Autodesk Inventor part; units mm, degrees
(part 4 of 4)
sketch "Sketch22" plane through (0, 0, 1.6) normal (0, 0, 1) x (1, 0, 0)
  line L0 (-10.5, 33.5) -> (-70.5, 33.5) projected
  line L1 (-70.5, 33.5) -> (-70.5, 17.8589) projected
  arc A0 (-71.1087, 16.5323) -> (-70.5, 17.8589) centre (-72.25, 17.8589) ccw projected
  arc A1 (-71.1087, 16.5323) -> (-71.1087, 10.4677) centre (-68.5, 13.5) ccw projected
  arc A2 (-70.5, 9.1411) -> (-71.1087, 10.4677) centre (-72.25, 9.1411) ccw projected
  line L2 (-70.5, 9.1411) -> (-70.5, 3) projected
  line L3 (-70.5, 3) -> (-53.1906, 3) projected
  line L4 (-53.1906, 3) -> (-51.7472, 0.5) projected
  arc A3 (-51.7472, -2.5) -> (-51.7472, 0.5) centre (-54.3453, -1) ccw projected
  line L5 (-51.7472, -2.5) -> (-53.1906, -5) projected
  line L6 (-53.1906, -5) -> (-70.5, -5) projected
  line L7 (-70.5, -5) -> (-70.5, -10.5) projected
  arc A4 (-71.3276, -12.569) -> (-70.5, -10.5) centre (-73.5, -10.5) ccw projected
  arc A5 (-71.3276, -12.569) -> (-71.3276, -28.431) centre (-63, -20.5) ccw projected
  arc A6 (-70.5, -30.5) -> (-71.3276, -28.431) centre (-73.5, -30.5) ccw projected
  line L8 (-70.5, -30.5) -> (-70.5, -37.5) projected
  line L9 (-70.5, -37.5) -> (-56.7679, -37.5) projected
  line L10 (-56.7679, -37.5) -> (-55.6132, -39.5) projected
  arc A7 (-55.6132, -41.5) -> (-55.6132, -39.5) centre (-57.3453, -40.5) ccw projected
  line L11 (-55.6132, -41.5) -> (-56.7679, -43.5) projected
  line L12 (-56.7679, -43.5) -> (-70.5, -43.5) projected
  line L13 (-70.5, -43.5) -> (-70.5, -47.4689) projected
  arc A8 (-70.5, -47.4689) -> (-69.0556, -48.3647) centre (-69.5, -47.4689) ccw projected
  arc A9 (-64.3647, -53.0556) -> (-69.0556, -48.3647) centre (-67.5, -51.5) ccw projected
  arc A10 (-64.3647, -53.0556) -> (-63.4689, -54.5) centre (-63.4689, -53.5) ccw projected
  line L14 (-63.4689, -54.5) -> (-47, -54.5) projected
  line L15 (-47, -54.5) -> (-47, -50) projected
  arc A11 (-45, -48) -> (-47, -50) centre (-45, -50) ccw projected
  line L16 (-45, -48) -> (24, -48) projected
  arc A12 (26, -50) -> (24, -48) centre (24, -50) ccw projected
  line L17 (26, -50) -> (26, -54.5) projected
  line L18 (26, -54.5) -> (63.4689, -54.5) projected
  arc A13 (63.4689, -54.5) -> (64.3647, -53.0556) centre (63.4689, -53.5) ccw projected
  arc A14 (69.0556, -48.3647) -> (64.3647, -53.0556) centre (67.5, -51.5) ccw projected
  arc A15 (69.0556, -48.3647) -> (70.5, -47.4689) centre (69.5, -47.4689) ccw projected
  line L19 (70.5, -47.4689) -> (70.5, -43.5) projected
  line L20 (70.5, -43.5) -> (57.2321, -43.5) projected
  line L21 (57.2321, -43.5) -> (58.5311, -41.25) projected
  arc A16 (58.5311, -41.25) -> (58.5311, -39.75) centre (57.2321, -40.5) ccw projected
  line L22 (58.5311, -39.75) -> (57.2321, -37.5) projected
  line L23 (57.2321, -37.5) -> (70.5, -37.5) projected
  line L24 (70.5, -37.5) -> (70.5, -30.5) projected
  arc A17 (71.3276, -28.431) -> (70.5, -30.5) centre (73.5, -30.5) ccw projected
  arc A18 (71.3276, -28.431) -> (71.3276, -12.569) centre (63, -20.5) ccw projected
  arc A19 (70.5, -10.5) -> (71.3276, -12.569) centre (73.5, -10.5) ccw projected
  line L25 (70.5, -10.5) -> (70.5, 9.6199) projected
  arc A20 (71, 10.9428) -> (70.5, 9.6199) centre (72.5, 9.6199) ccw projected
  arc A21 (71, 10.9428) -> (72.25, 14.25) centre (67.25, 14.25) ccw projected
  line L26 (72.25, 14.25) -> (72.25, 43.95) projected
  arc A22 (72.25, 43.95) -> (71, 47.2572) centre (67.25, 43.95) ccw projected
  arc A23 (70.6186, 47.9015) -> (71, 47.2572) centre (72.5, 48.5801) ccw projected
  arc A24 (70.6186, 47.9015) -> (69.194, 48.4372) centre (69.678, 47.5622) ccw projected
  arc A25 (64.3647, 53.0556) -> (69.194, 48.4372) centre (67.5, 51.5) ccw projected
  arc A26 (64.3647, 53.0556) -> (63.4689, 54.5) centre (63.4689, 53.5) ccw projected
  line L27 (63.4689, 54.5) -> (-63.4689, 54.5) projected
  arc A27 (-63.4689, 54.5) -> (-64.3647, 53.0556) centre (-63.4689, 53.5) ccw projected
  arc A28 (-69.0556, 48.3647) -> (-64.3647, 53.0556) centre (-67.5, 51.5) ccw projected
  arc A29 (-69.0556, 48.3647) -> (-70.5, 47.4689) centre (-69.5, 47.4689) ccw projected
  line L28 (-70.5, 47.4689) -> (-70.5, 39.5) projected
  line L29 (-70.5, 39.5) -> (-10.5, 39.5) projected
  arc A30 (-10.5, 33.5) -> (-10.5, 39.5) centre (-10.5, 36.5) ccw projected
  line L30 (33.5, 22.1) -> (33.5, 39.1) projected
  arc A31 (33.9581, 40.3738) -> (33.5, 39.1) centre (35.5, 39.1) ccw projected
  arc A32 (33.9581, 40.3738) -> (34.4469, 40.1682) centre (35.75, 43.95) ccw projected
  arc A33 (34.4469, 40.1682) -> (34, 39.1) centre (35.5, 39.1) ccw projected
  line L31 (34, 39.1) -> (34, 22.1) projected
  arc A34 (34, 22.1) -> (35.5, 20.6) centre (35.5, 22.1) ccw projected
  line L32 (35.5, 20.6) -> (67.5, 20.6) projected
  arc A35 (67.5, 20.6) -> (69, 22.1) centre (67.5, 22.1) ccw projected
  line L33 (69, 22.1) -> (69, 39.1) projected
  arc A36 (69, 39.1) -> (68.5531, 40.1682) centre (67.5, 39.1) ccw projected
  arc A37 (68.5531, 40.1682) -> (69.0419, 40.3738) centre (67.25, 43.95) ccw projected
  arc A38 (69.5, 39.1) -> (69.0419, 40.3738) centre (67.5, 39.1) ccw projected
  line L34 (69.5, 39.1) -> (69.5, 22.1) projected
  arc A39 (67.5, 20.1) -> (69.5, 22.1) centre (67.5, 22.1) ccw projected
  line L35 (67.5, 20.1) -> (35.5, 20.1) projected
  arc A40 (33.5, 22.1) -> (35.5, 20.1) centre (35.5, 22.1) ccw projected
  arc A41 (70.5, 39.1) -> (69.8755, 40.9322) centre (67.5, 39.1) ccw projected
  line L36 (70.5, 39.1) -> (70.5, 22.1) projected
  arc A42 (67.5, 19.1) -> (70.5, 22.1) centre (67.5, 22.1) ccw projected
  line L37 (67.5, 19.1) -> (35.5, 19.1) projected
  arc A43 (32.5, 22.1) -> (35.5, 19.1) centre (35.5, 22.1) ccw projected
  line L38 (32.5, 22.1) -> (32.5, 39.1) projected
  arc A44 (33.1245, 40.9322) -> (32.5, 39.1) centre (35.5, 39.1) ccw projected
  arc A45 (33.1245, 40.9322) -> (33.5215, 40.6283) centre (35.75, 43.95) ccw projected
  arc A46 (33.5215, 40.6283) -> (33, 39.1) centre (35.5, 39.1) ccw projected
  line L39 (33, 39.1) -> (33, 22.1) projected
  arc A47 (33, 22.1) -> (35.5, 19.6) centre (35.5, 22.1) ccw projected
  line L40 (35.5, 19.6) -> (67.5, 19.6) projected
  arc A48 (67.5, 19.6) -> (70, 22.1) centre (67.5, 22.1) ccw projected
  line L41 (70, 22.1) -> (70, 39.1) projected
  arc A49 (70, 39.1) -> (69.4785, 40.6283) centre (67.5, 39.1) ccw projected
  arc A50 (69.4785, 40.6283) -> (69.8755, 40.9322) centre (67.25, 43.95) ccw projected
  arc A51 (37.9357, 40.6) -> (38.5567, 41.1) centre (35.75, 43.95) ccw projected
  line L42 (38.5567, 41.1) -> (64.4433, 41.1) projected
  arc A52 (64.4433, 41.1) -> (65.0643, 40.6) centre (67.25, 43.95) ccw projected
  line L43 (65.0643, 40.6) -> (37.9357, 40.6) projected
  arc A53 (63.7035, 42.1) -> (64.0131, 41.6) centre (67.25, 43.95) ccw projected
  line L44 (64.0131, 41.6) -> (38.9869, 41.6) projected
  arc A54 (38.9869, 41.6) -> (39.2965, 42.1) centre (35.75, 43.95) ccw projected
  line L45 (39.2965, 42.1) -> (63.7035, 42.1) projected
  line L46 (49, -24.373) -> (49, -33.5) projected
  arc A55 (47, -35.5) -> (49, -33.5) centre (47, -33.5) ccw projected
  line L47 (47, -35.5) -> (37, -35.5) projected
  arc A56 (35, -33.5) -> (37, -35.5) centre (37, -33.5) ccw projected
  line L48 (35, -33.5) -> (35, -24.373) projected
  arc A57 (37, -14.255) -> (35, -24.373) centre (42, -20.5) ccw projected
  line L49 (37, -14.255) -> (37, -6) projected
  arc A58 (47, -6) -> (37, -6) centre (42, -6) ccw projected
  line L50 (47, -6) -> (47, -14.255) projected
  arc A59 (49, -24.373) -> (47, -14.255) centre (42, -20.5) ccw projected
  line L51 (34.5, 22.1) -> (34.5, 39.1) projected
  arc A60 (35.5, 40.1) -> (34.5, 39.1) centre (35.5, 39.1) ccw projected
  line L52 (35.5, 40.1) -> (67.5, 40.1) projected
  arc A61 (68.5, 39.1) -> (67.5, 40.1) centre (67.5, 39.1) ccw projected
  line L53 (68.5, 39.1) -> (68.5, 22.1) projected
  arc A62 (67.5, 21.1) -> (68.5, 22.1) centre (67.5, 22.1) ccw projected
  line L54 (67.5, 21.1) -> (35.5, 21.1) projected
  arc A63 (34.5, 22.1) -> (35.5, 21.1) centre (35.5, 22.1) ccw projected
  circle A64 centre (35.75, 43.95) radius 3 projected
  circle A65 centre (67.25, 43.95) radius 3 projected
  circle A66 centre (67.25, 14.25) radius 3 projected
  circle A67 centre (35.75, 14.25) radius 3 projected
  circle A68 centre (-31.5, -14) radius 3.5 projected
  circle A69 centre (31.5, -14) radius 3.5 projected
  circle A70 centre (-10.5, -14) radius 3.5 projected
  circle A71 centre (10.5, -14) radius 3.5 projected
  line L55 (-47, -33.5) -> (-47, -26.745) projected
  arc A72 (-47, -14.255) -> (-47, -26.745) centre (-42, -20.5) ccw projected
  line L56 (-47, -14.255) -> (-47, -6) projected
  arc A73 (-37, -6) -> (-47, -6) centre (-42, -6) ccw projected
  line L57 (-37, -6) -> (-37, -14.255) projected
  arc A74 (-37, -26.745) -> (-37, -14.255) centre (-42, -20.5) ccw projected
  line L58 (-37, -26.745) -> (-37, -33.5) projected
  arc A75 (-39, -35.5) -> (-37, -33.5) centre (-39, -33.5) ccw projected
  line L59 (-39, -35.5) -> (-45, -35.5) projected
  arc A76 (-47, -33.5) -> (-45, -35.5) centre (-45, -33.5) ccw projected
  line L60 (-26, -33.5) -> (-26, -26.745) projected
  arc A77 (-26, -14.255) -> (-26, -26.745) centre (-21, -20.5) ccw projected
  line L61 (-26, -14.255) -> (-26, -6) projected
  arc A78 (-16, -6) -> (-26, -6) centre (-21, -6) ccw projected
  line L62 (-16, -6) -> (-16, -14.255) projected
  arc A79 (-16, -26.745) -> (-16, -14.255) centre (-21, -20.5) ccw projected
  line L63 (-16, -26.745) -> (-16, -33.5) projected
  arc A80 (-18, -35.5) -> (-16, -33.5) centre (-18, -33.5) ccw projected
  line L64 (-18, -35.5) -> (-24, -35.5) projected
  arc A81 (-26, -33.5) -> (-24, -35.5) centre (-24, -33.5) ccw projected
  line L65 (-5, -33.5) -> (-5, -26.745) projected
  arc A82 (-5, -14.255) -> (-5, -26.745) centre (0, -20.5) ccw projected
  line L66 (-5, -14.255) -> (-5, -6) projected
  arc A83 (5, -6) -> (-5, -6) centre (0, -6) ccw projected
  line L67 (5, -6) -> (5, -14.255) projected
  arc A84 (5, -26.745) -> (5, -14.255) centre (0, -20.5) ccw projected
  line L68 (5, -26.745) -> (5, -33.5) projected
  arc A85 (3, -35.5) -> (5, -33.5) centre (3, -33.5) ccw projected
  line L69 (3, -35.5) -> (-3, -35.5) projected
  arc A86 (-5, -33.5) -> (-3, -35.5) centre (-3, -33.5) ccw projected
  line L70 (16, -33.5) -> (16, -26.745) projected
  arc A87 (16, -14.255) -> (16, -26.745) centre (21, -20.5) ccw projected
  line L71 (16, -14.255) -> (16, -6) projected
  arc A88 (26, -6) -> (16, -6) centre (21, -6) ccw projected
  line L72 (26, -6) -> (26, -14.255) projected
  arc A89 (26, -26.745) -> (26, -14.255) centre (21, -20.5) ccw projected
  line L73 (26, -26.745) -> (26, -33.5) projected
  arc A90 (24, -35.5) -> (26, -33.5) centre (24, -33.5) ccw projected
  line L74 (24, -35.5) -> (18, -35.5) projected
  arc A91 (16, -33.5) -> (18, -35.5) centre (18, -33.5) ccw projected
  arc A92 (58, -6.5) -> (56, -8.5) centre (58, -8.5) ccw projected
  line L75 (58, -6.5) -> (70, -6.5) projected
  line L76 (70, -6.5) -> (70, -10.5) projected
  arc A93 (70, -10.5) -> (70.9655, -12.9138) centre (73.5, -10.5) ccw projected
  arc A94 (55.0345, -12.9138) -> (70.9655, -12.9138) centre (63, -20.5) ccw projected
  arc A95 (55.0345, -12.9138) -> (56, -10.5) centre (52.5, -10.5) ccw projected
  line L77 (56, -10.5) -> (56, -8.5) projected
  arc A96 (-58, -34.5) -> (-56, -32.5) centre (-58, -32.5) ccw projected
  line L78 (-58, -34.5) -> (-70, -34.5) projected
  line L79 (-70, -34.5) -> (-70, -30.5) projected
  arc A97 (-70, -30.5) -> (-70.9655, -28.0862) centre (-73.5, -30.5) ccw projected
  arc A98 (-55.0345, -28.0862) -> (-70.9655, -28.0862) centre (-63, -20.5) ccw projected
  arc A99 (-55.0345, -28.0862) -> (-56, -30.5) centre (-52.5, -30.5) ccw projected
  line L80 (-56, -30.5) -> (-56, -32.5) projected
  line L81 (-53.5, 10) -> (-68.5, 10) projected
  arc A100 (-70.7826, 16.1532) -> (-68.5, 10) centre (-68.5, 13.5) ccw projected
  arc A101 (-70.7826, 16.1532) -> (-70, 17.8589) centre (-72.25, 17.8589) ccw projected
  line L82 (-70, 17.8589) -> (-70, 22) projected
  line L83 (-70, 22) -> (-54, 22) projected
  arc A102 (-52, 20) -> (-54, 22) centre (-54, 20) ccw projected
  line L84 (-52, 20) -> (-52, 17.8589) projected
  arc A103 (-52, 17.8589) -> (-51.2174, 16.1532) centre (-49.75, 17.8589) ccw projected
  arc A104 (-53.5, 10) -> (-51.2174, 16.1532) centre (-53.5, 13.5) ccw projected
  line L85 (-48, -6) -> (-48, -13.7918)
  arc A105 (-48, -13.7918) -> (-48, -27.2082) centre (-42, -20.5) ccw
  line L86 (-48, -27.2082) -> (-48, -33.5)
  arc A106 (-48, -33.5) -> (-45, -36.5) centre (-45, -33.5) ccw
  line L87 (-45, -36.5) -> (-39, -36.5)
  arc A107 (-39, -36.5) -> (-36, -33.5) centre (-39, -33.5) ccw
  line L88 (-36, -33.5) -> (-36, -27.2082)
  arc A108 (-36, -27.2082) -> (-36, -13.7918) centre (-42, -20.5) ccw
  line L89 (-36, -13.7918) -> (-36, -6)
  arc A109 (-36, -6) -> (-48, -6) centre (-42, -6) ccw
  line L90 (-27, -6) -> (-27, -13.7918)
  arc A110 (-27, -13.7918) -> (-27, -27.2082) centre (-21, -20.5) ccw
  line L91 (-27, -27.2082) -> (-27, -33.5)
  arc A111 (-27, -33.5) -> (-24, -36.5) centre (-24, -33.5) ccw
  line L92 (-24, -36.5) -> (-18, -36.5)
  arc A112 (-18, -36.5) -> (-15, -33.5) centre (-18, -33.5) ccw
  line L93 (-15, -33.5) -> (-15, -27.2082)
  arc A113 (-15, -27.2082) -> (-15, -13.7918) centre (-21, -20.5) ccw
  line L94 (-15, -13.7918) -> (-15, -6)
  arc A114 (-15, -6) -> (-27, -6) centre (-21, -6) ccw
  line L95 (-6, -6) -> (-6, -13.7918)
  arc A115 (-6, -13.7918) -> (-6, -27.2082) centre (0, -20.5) ccw
  line L96 (-6, -27.2082) -> (-6, -33.5)
  arc A116 (-6, -33.5) -> (-3, -36.5) centre (-3, -33.5) ccw
  line L97 (-3, -36.5) -> (3, -36.5)
  arc A117 (3, -36.5) -> (6, -33.5) centre (3, -33.5) ccw
  line L98 (6, -33.5) -> (6, -27.2082)
  arc A118 (6, -27.2082) -> (6, -13.7918) centre (0, -20.5) ccw
  line L99 (6, -13.7918) -> (6, -6)
  arc A119 (6, -6) -> (-6, -6) centre (0, -6) ccw
  line L100 (15, -6) -> (15, -13.7918)
  arc A120 (15, -13.7918) -> (15, -27.2082) centre (21, -20.5) ccw
  line L101 (15, -27.2082) -> (15, -33.5)
  arc A121 (15, -33.5) -> (18, -36.5) centre (18, -33.5) ccw
  line L102 (18, -36.5) -> (24, -36.5)
  arc A122 (24, -36.5) -> (27, -33.5) centre (24, -33.5) ccw
  line L103 (27, -33.5) -> (27, -27.2082)
  arc A123 (27, -27.2082) -> (27, -13.7918) centre (21, -20.5) ccw
  line L104 (27, -13.7918) -> (27, -6)
  arc A124 (27, -6) -> (15, -6) centre (21, -6) ccw
  line L105 (-70.5, 54.5) -> (-6.5, 54.5)
  line L106 (-6.5, 54.5) -> (-6.5, 36.5)
  line L107 (-10.5, 32.5) -> (-70.5, 32.5)
  line L108 (-70.5, 32.5) -> (-70.5, 54.5)
  line L109 (-63.4689, 54.5) -> (63.4689, 54.5) projected
  line L110 (-70.5, 39.5) -> (-70.5, 47.4689) projected
  arc A125 (-10.5, 32.5) -> (-6.5, 36.5) centre (-10.5, 36.5) ccw
  arc A126 (-10.5, 33.5) -> (-10.5, 39.5) centre (-10.5, 36.5) ccw projected
  point P0 (0, 0)
  point P1 (13.8395, -15.0477)
  point P2 (12.9269, -16.5219)
  point P3 (29.0731, -16.5219)
  point P4 (28.1605, -15.0477)
  point P5 (-7.1605, -15.0477)
  point P6 (-8.0731, -16.5219)
  point P7 (8.0731, -16.5219)
  point P8 (7.1605, -15.0477)
  point P9 (-28.1605, -15.0477)
  point P10 (-29.0731, -16.5219)
  point P11 (-12.9269, -16.5219)
  point P12 (-13.8395, -15.0477)
  point P13 (-33.9269, -16.5219)
  point P14 (-34.8395, -15.0477)
  point P15 (-6.5, 54.5)
  dimension "d180" = 1
  dimension "d181" = 1
  dimension "d182" = 1
  dimension "d183" = 1
  dimension "d184" = 1
  constraints: 48 end point, 42 point on circle, 21 centre point, 2 collinear, 2 parallel, 2 tangent, 1 concentric, 1 horizontal, 1 perpendicular, 36 other
  measures "d180" radial gap between concentric circles of A73 A109
  measures "d181" radial gap between concentric circles of A78 A114
  measures "d182" radial gap between concentric circles of A83 A119
  measures "d183" radial gap between concentric circles of A88 A124
  measures "d184" distance between parallel lines of L107 L0
sketch "Sketch15" plane through (0, 0, 1.6) normal (0, 0, 1) x (1, 0, 0)
  line L0 (-47, -54.5) -> (-47, -50) projected
  arc A0 (-45, -48) -> (-47, -50) centre (-45, -50) ccw projected
  line L1 (-45, -48) -> (24, -48) projected
  arc A1 (26, -50) -> (24, -48) centre (24, -50) ccw projected
  line L2 (26, -50) -> (26, -54.5) projected
  line L3 (26, -54.5) -> (63.4689, -54.5) projected
  arc A2 (63.4689, -54.5) -> (64.3647, -53.0556) centre (63.4689, -53.5) ccw projected
  arc A3 (69.0556, -48.3647) -> (70.5, -47.4689) centre (69.5, -47.4689) ccw projected
  arc A4 (64.3647, 53.0556) -> (63.4689, 54.5) centre (63.4689, 53.5) ccw projected
  line L4 (63.4689, 54.5) -> (-63.4689, 54.5) projected
  arc A5 (-63.4689, 54.5) -> (-64.3647, 53.0556) centre (-63.4689, 53.5) ccw projected
  arc A6 (-69.0556, 48.3647) -> (-70.5, 47.4689) centre (-69.5, 47.4689) ccw projected
  arc A7 (-70.5, -47.4689) -> (-69.0556, -48.3647) centre (-69.5, -47.4689) ccw projected
  arc A8 (-64.3647, -53.0556) -> (-63.4689, -54.5) centre (-63.4689, -53.5) ccw projected
  line L5 (-63.4689, -54.5) -> (-47, -54.5) projected
  circle A9 centre (35.75, 14.25) radius 3 projected
  circle A10 centre (67.25, 14.25) radius 3 projected
  circle A11 centre (67.25, 43.95) radius 3 projected
  circle A12 centre (35.75, 43.95) radius 3 projected
  line L6 (34.5, 22.1) -> (34.5, 39.1) projected
  arc A13 (35.5, 40.1) -> (34.5, 39.1) centre (35.5, 39.1) ccw projected
  line L7 (35.5, 40.1) -> (67.5, 40.1) projected
  arc A14 (68.5, 39.1) -> (67.5, 40.1) centre (67.5, 39.1) ccw projected
  line L8 (68.5, 39.1) -> (68.5, 22.1) projected
  arc A15 (67.5, 21.1) -> (68.5, 22.1) centre (67.5, 22.1) ccw projected
  line L9 (67.5, 21.1) -> (35.5, 21.1) projected
  arc A16 (34.5, 22.1) -> (35.5, 21.1) centre (35.5, 22.1) ccw projected
  circle A17 centre (-53.5, 13.5) radius 1.7 projected
  circle A18 centre (-58.5, 13.5) radius 1.7 projected
  circle A19 centre (-63.5, 13.5) radius 1.7 projected
  circle A20 centre (-68.5, 13.5) radius 1.7 projected
  circle A21 centre (63, -20.5) radius 8 projected
  circle A22 centre (-63, -20.5) radius 8 projected
  line L10 (-47, -33.5) -> (-47, -26.745) projected
  arc A23 (-47, -14.255) -> (-47, -26.745) centre (-42, -20.5) ccw projected
  line L11 (-47, -14.255) -> (-47, -6) projected
  arc A24 (-37, -6) -> (-47, -6) centre (-42, -6) ccw projected
  line L12 (-37, -6) -> (-37, -14.255) projected
  arc A25 (-37, -26.745) -> (-37, -14.255) centre (-42, -20.5) ccw projected
  line L13 (-37, -26.745) -> (-37, -33.5) projected
  arc A26 (-39, -35.5) -> (-37, -33.5) centre (-39, -33.5) ccw projected
  line L14 (-39, -35.5) -> (-45, -35.5) projected
  arc A27 (-47, -33.5) -> (-45, -35.5) centre (-45, -33.5) ccw projected
  line L15 (-26, -33.5) -> (-26, -26.745) projected
  arc A28 (-26, -14.255) -> (-26, -26.745) centre (-21, -20.5) ccw projected
  line L16 (-26, -14.255) -> (-26, -6) projected
  arc A29 (-16, -6) -> (-26, -6) centre (-21, -6) ccw projected
  line L17 (-16, -6) -> (-16, -14.255) projected
  arc A30 (-16, -26.745) -> (-16, -14.255) centre (-21, -20.5) ccw projected
  line L18 (-16, -26.745) -> (-16, -33.5) projected
  arc A31 (-18, -35.5) -> (-16, -33.5) centre (-18, -33.5) ccw projected
  line L19 (-18, -35.5) -> (-24, -35.5) projected
  arc A32 (-26, -33.5) -> (-24, -35.5) centre (-24, -33.5) ccw projected
  line L20 (-5, -33.5) -> (-5, -26.745) projected
  arc A33 (-5, -14.255) -> (-5, -26.745) centre (0, -20.5) ccw projected
  line L21 (-5, -14.255) -> (-5, -6) projected
  arc A34 (5, -6) -> (-5, -6) centre (0, -6) ccw projected
  line L22 (5, -6) -> (5, -14.255) projected
  arc A35 (5, -26.745) -> (5, -14.255) centre (0, -20.5) ccw projected
  line L23 (5, -26.745) -> (5, -33.5) projected
  arc A36 (3, -35.5) -> (5, -33.5) centre (3, -33.5) ccw projected
  line L24 (3, -35.5) -> (-3, -35.5) projected
  arc A37 (-5, -33.5) -> (-3, -35.5) centre (-3, -33.5) ccw projected
  line L25 (16, -33.5) -> (16, -26.745) projected
  arc A38 (16, -14.255) -> (16, -26.745) centre (21, -20.5) ccw projected
  line L26 (16, -14.255) -> (16, -6) projected
  arc A39 (26, -6) -> (16, -6) centre (21, -6) ccw projected
  line L27 (26, -6) -> (26, -14.255) projected
  arc A40 (26, -26.745) -> (26, -14.255) centre (21, -20.5) ccw projected
  line L28 (26, -26.745) -> (26, -33.5) projected
  arc A41 (24, -35.5) -> (26, -33.5) centre (24, -33.5) ccw projected
  line L29 (24, -35.5) -> (18, -35.5) projected
  arc A42 (16, -33.5) -> (18, -35.5) centre (18, -33.5) ccw projected
  line L30 (35, -33.5) -> (35, -24.373) projected
  arc A43 (37, -14.255) -> (35, -24.373) centre (42, -20.5) ccw projected
  line L31 (37, -14.255) -> (37, -6) projected
  arc A44 (47, -6) -> (37, -6) centre (42, -6) ccw projected
  line L32 (47, -6) -> (47, -14.255) projected
  arc A45 (49, -24.373) -> (47, -14.255) centre (42, -20.5) ccw projected
  line L33 (49, -24.373) -> (49, -33.5) projected
  arc A46 (47, -35.5) -> (49, -33.5) centre (47, -33.5) ccw projected
  line L34 (47, -35.5) -> (37, -35.5) projected
  arc A47 (35, -33.5) -> (37, -35.5) centre (37, -33.5) ccw projected
  circle A48 centre (63, -20.5) radius 11
  line L35 (63, -31.5) -> (70.5, -31.5)
  line L36 (70.5, -29.7376) -> (70.5, -47.4689) projected
  line L37 (70.5, -5.5) -> (57.5, -5.5)
  line L38 (55.5, -7.5) -> (55.5, -12.4533)
  line L39 (55.5, -12.4533) -> (70.5, -12.4533)
  line L40 (70.5, -12.4533) -> (70.5, -5.5)
  arc A49 (57.5, -5.5) -> (55.5, -7.5) centre (57.5, -7.5) ccw
  arc A50 (47, -35.5) -> (49, -33.5) centre (47, -33.5) ccw projected
  line L41 (55.5, -7.5) -> (70.5, -7.5) construction
  arc A51 (69.0556, -48.3647) -> (64.3647, -53.0556) centre (67.5, -51.5) ccw projected
  line L42 (70.5, -47.4689) -> (70.5, -29.7601) projected
  arc A52 (71.25, -27.7758) -> (70.5, -29.7601) centre (73.5, -29.7601) ccw projected
  arc A53 (71.25, -27.7758) -> (71.25, -13.2242) centre (63, -20.5) ccw projected
  arc A54 (70.5, -11.2399) -> (71.25, -13.2242) centre (73.5, -11.2399) ccw projected
  line L43 (70.5, -11.2399) -> (70.5, 9.6199) projected
  arc A55 (71, 10.9428) -> (70.5, 9.6199) centre (72.5, 9.6199) ccw projected
  arc A56 (71, 10.9428) -> (72.25, 14.25) centre (67.25, 14.25) ccw projected
  line L44 (72.25, 14.25) -> (72.25, 43.95) projected
  arc A57 (72.25, 43.95) -> (71, 47.2572) centre (67.25, 43.95) ccw projected
  arc A58 (70.6186, 47.9015) -> (71, 47.2572) centre (72.5, 48.5801) ccw projected
  arc A59 (70.6186, 47.9015) -> (69.194, 48.4372) centre (69.678, 47.5622) ccw projected
  arc A60 (64.3647, 53.0556) -> (69.194, 48.4372) centre (67.5, 51.5) ccw projected
  arc A61 (-69.0556, 48.3647) -> (-64.3647, 53.0556) centre (-67.5, 51.5) ccw projected
  line L45 (-70.5, 47.4689) -> (-70.5, 17.8589) projected
  arc A62 (-71.1087, 16.5323) -> (-70.5, 17.8589) centre (-72.25, 17.8589) ccw projected
  arc A63 (-71.1087, 16.5323) -> (-71.1087, 10.4677) centre (-68.5, 13.5) ccw projected
  arc A64 (-70.5, 9.1411) -> (-71.1087, 10.4677) centre (-72.25, 9.1411) ccw projected
  line L46 (-70.5, 9.1411) -> (-70.5, -11.2399) projected
  arc A65 (-71.25, -13.2242) -> (-70.5, -11.2399) centre (-73.5, -11.2399) ccw projected
  arc A66 (-71.25, -13.2242) -> (-71.25, -27.7758) centre (-63, -20.5) ccw projected
  arc A67 (-70.5, -29.7601) -> (-71.25, -27.7758) centre (-73.5, -29.7601) ccw projected
  line L47 (-70.5, -29.7601) -> (-70.5, -47.4689) projected
  arc A68 (-64.3647, -53.0556) -> (-69.0556, -48.3647) centre (-67.5, -51.5) ccw projected
  point P0 (0, 0)
  point P1 (55.5, -5.5)
  point P2 (63, -7.5)
  dimension "d118" = 22
  dimension "d120" = 4
  constraints: 12 end point, 4 point on circle, 4 point on line, 3 tangent, 2 centre point, 2 horizontal, 2 parallel, 2 perpendicular, 1 coincident, 1 equal radius, 1 midpoint, 1 vertical alignment
  measures "d118" diameter of A48
  measures "d120" distance edge to line of A48 L37
equation "\"d9\" = d8"
equation "\"d8\" = 21"
body "Solid1"
